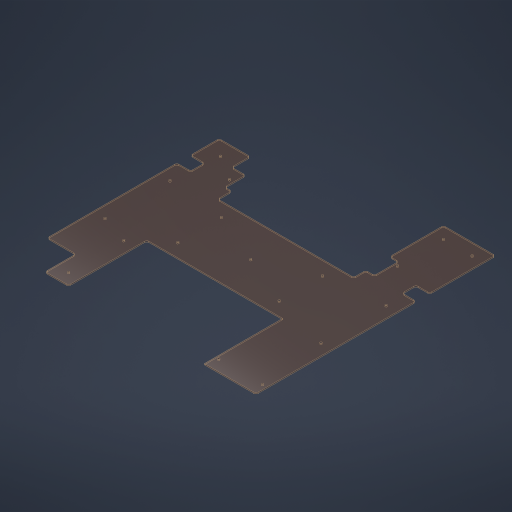
# Autodesk Inventor part: DB1-023
Saved by Autodesk Inventor 2023.4 (Build 274418000, 418)
## iProperties
Created: 2025-03-10
Part Number: DB1-023
Material: Polycarbonate, Smoke
Document SubType Name: Sheet Metal
Designer: brand
Density: 1.2 g/cm^3
Sheet Metal Rule: Default
Appearance: Polycarbonate - Smoked
Author: brand
Autodesk Inventor part; units mm, degrees
ref_plane "YZ Plane" through (0, 0, 0) normal (1, 0, 0) x (0, 1, 0)
ref_plane "XZ Plane" through (0, 0, 0) normal (0, 1, 0) x (-1, 0, 0)
ref_plane "XY Plane" through (0, 0, 0) normal (0, 0, 1) x (1, 0, 0)
sketch "Sketch1" plane through (0, 0, 0) normal (0, 1, 0) x (-1, 0, 0)
  line L0 (329.819, 329.819) -> (-329.819, 329.819)
  line L1 (-329.819, 329.819) -> (-329.819, -329.819)
  line L2 (-329.819, -329.819) -> (329.819, -329.819)
  line L3 (329.819, -329.819) -> (329.819, 329.819)
  line L4 (329.819, 329.819) -> (-329.819, -329.819) construction
  line L5 (-329.819, 329.819) -> (329.819, -329.819) construction
  line L6 (187.325, 329.819) -> (-187.325, 329.819) construction
  line L7 (-187.325, 329.819) -> (-187.325, 113.919)
  line L8 (-187.325, 113.919) -> (187.325, 113.919)
  line L9 (187.325, 113.919) -> (187.325, 329.819)
  line L10 (187.325, -329.819) -> (-187.325, -329.819) construction
  line L11 (-187.325, -329.819) -> (-187.325, -82.169)
  line L12 (-187.325, -82.169) -> (187.325, -82.169)
  line L13 (187.325, -82.169) -> (187.325, -329.819)
  point P0 (0, 0)
  point P1 (0, 329.819)
  point P2 (0, 329.819)
  point P3 (0, -329.819)
  point P4 (0, -329.819)
  point P5 (-187.325, 329.819)
  dimension "d0" = 659.638
  dimension "d1" = 659.638
  dimension "d3" = 215.9
  dimension "d4" = 247.65
  dimension "d5" = 374.65
  constraints: 28 end point, 6 midpoint, 6 parallel, 3 horizontal, 3 perpendicular, 2 coincident, 2 point on line, 1 collinear
  measures "d0" distance of L0.start L0.end
  measures "d1" distance of L2.end L0.start
  measures "d3" distance of L8.end L6.start
  measures "d4" distance of L12.end L10.start
  measures "d5" distance of L11.end L12.end
extrude "Extrusion1" add sketch "Sketch1" along normal mid plane 3.175 contours L3 L2 L13 L12 L11 L1 L0 L7 L8 L9
sketch "Sketch2" plane through (0, 1.5875, 0) normal (0, 1, 0) x (1, 0, 0)
  circle A0 centre (-283.3124, 275.8316) radius 34.925 construction
  line L0 (329.819, 329.819) -> (329.819, -329.819) construction
  line L1 (329.819, -329.819) -> (187.325, -329.819) construction
  line L2 (187.325, -329.819) -> (187.325, -113.919) construction
  line L3 (187.325, -113.919) -> (-187.325, -113.919) construction
  line L4 (-187.325, -113.919) -> (-187.325, -329.819) construction
  line L5 (-187.325, -329.819) -> (-329.819, -329.819) construction
  line L6 (-329.819, -329.819) -> (-329.819, 329.819) construction
  line L7 (-329.819, 329.819) -> (-187.325, 329.819) construction
  line L8 (-187.325, 329.819) -> (-187.325, 82.169) construction
  line L9 (-187.325, 82.169) -> (187.325, 82.169) construction
  line L10 (187.325, 82.169) -> (187.325, 329.819) construction
  line L11 (187.325, 329.819) -> (329.819, 329.819) construction
  line L12 (-187.325, 329.819) -> (-329.819, 329.819) construction
  line L13 (-329.819, 329.819) -> (-187.325, 329.819)
  line L14 (-187.325, 329.819) -> (-187.325, 228.219)
  line L15 (-187.325, 228.219) -> (-329.819, 228.219)
  line L16 (-329.819, 228.219) -> (-329.819, 329.819)
  line L17 (329.819, -329.819) -> (187.325, -329.819) construction
  line L18 (187.325, -113.919) -> (206.375, -113.919)
  line L19 (206.375, -113.919) -> (206.375, -329.819)
  line L20 (206.375, -329.819) -> (187.325, -329.819)
  line L21 (187.325, -329.819) -> (187.325, -113.919)
  line L22 (-329.819, 329.819) -> (-329.819, -329.819) construction
  line L23 (-329.819, 149.606) -> (-291.719, 149.606)
  line L24 (-291.719, 149.606) -> (-291.719, 111.506)
  line L25 (-291.719, 111.506) -> (-329.819, 111.506)
  line L26 (-329.819, 111.506) -> (-329.819, 149.606)
  line L27 (329.819, 149.606) -> (291.719, 149.606)
  line L28 (291.719, 149.606) -> (291.719, 111.506)
  line L29 (291.719, 111.506) -> (329.819, 111.506)
  line L30 (329.819, 111.506) -> (329.819, 149.606)
  line L31 (206.375, -113.919) -> (250.825, -113.919)
  line L32 (250.825, -113.919) -> (250.825, -266.319)
  line L33 (250.825, -266.319) -> (206.375, -266.319)
  line L34 (206.375, -266.319) -> (206.375, -113.919)
  line L35 (-187.325, 82.169) -> (-187.325, 329.819) construction
  line L36 (-187.325, 228.219) -> (-244.475, 228.219)
  line L37 (-244.475, 228.219) -> (-244.475, 177.419)
  line L38 (-244.475, 177.419) -> (-187.325, 177.419)
  line L39 (-187.325, 177.419) -> (-187.325, 228.219)
  circle A1 centre (-219.075, 209.169) radius 19.05 construction
  line L40 (-329.819, -329.819) -> (-187.325, -329.819) construction
  line L41 (-329.819, -329.819) -> (-187.325, -329.819)
  line L42 (-187.325, -329.819) -> (-187.325, -228.219)
  line L43 (-187.325, -228.219) -> (-329.819, -228.219)
  line L44 (-329.819, -228.219) -> (-329.819, -329.819)
  point P0 (0, 0)
  point P1 (-329.819, 130.556)
  dimension "d9" = 69.85
  dimension "d10" = 46.5066
  dimension "d11" = 53.9874
  dimension "d12" = 101.6
  dimension "d16" = 19.05
  dimension "d17" = 460.375
  dimension "d18" = 38.1
  dimension "d19" = 38.1
  dimension "d20" = 63.5
  dimension "d21" = 63.5
  dimension "d28" = 38.1
  dimension "d29" = 31.75
  dimension "d30" = 120.65
  dimension "d31" = 57.15
  dimension "d32" = 50.8
  dimension "d61" = 101.6
  constraints: 56 end point, 15 parallel, 7 horizontal, 7 perpendicular, 5 point on line, 2 centre point, 2 horizontal alignment, 1 midpoint
  measures "d9" diameter of A0
  measures "d10" distance from line of L16 A0.centre
  measures "d11" distance from line of L7 A0.centre
  measures "d12" distance of L13.end L14.end
  measures "d16" distance of L2.end L18.end
  measures "d17" distance from line of L5 point (-329.819, 130.556)
  measures "d18" distance of L23.end L24.end
  measures "d19" distance of L24.end L25.end
  measures "d20" distance between parallel lines of L2 L32
  measures "d21" distance between parallel lines of L1 L33
  measures "d28" diameter of A1
  measures "d29" distance from line of L35 A1.centre
  measures "d30" distance from line of L7 A1.centre
  measures "d31" distance of L37.end L38.end
  measures "d32" distance of L36.end L37.end
  measures "d61" distance of L43.end L5.end
extrude "Extrusion2" cut sketch "Sketch2" against normal through all contours L13 L14 L15 L16 | L39 L38 L37 L15 | L23 L24 L25 L26 | L30 L29 L28 L27
fillet "Fillet1" radius 5.715 20 edges at (-187.325, 0, 113.919) (329.819, 0, 329.819) (329.819, 0, -329.819) (187.325, 0, -329.819) (187.325, 0, -82.169) (-187.325, 0, -82.169) (-329.819, 0, 329.819) (-329.819, 0, -228.219) (-329.819, 0, -149.606) (-291.719, 0, -149.606) (-291.719, 0, -111.506) (-329.819, 0, -111.506) (291.719, 0, -149.606) (291.719, 0, -111.506) (329.819, 0, -111.506) (329.819, 0, -149.606) (-187.325, 0, -177.419) (-244.475, 0, -177.419) (-244.475, 0, -228.219) (-187.325, 0, 329.819)
sketch "Sketch4" plane through (0, 1.5875, 0) normal (0, 1, 0) x (1, 0, 0)
  arc A0 (324.104, -329.819) -> (329.819, -324.104) centre (324.104, -324.104) ccw construction
  line L0 (324.104, -329.819) -> (187.325, -329.819) construction
  line L1 (187.325, -113.919) -> (-181.61, -113.919) construction
  arc A1 (-181.61, -113.919) -> (-187.325, -119.634) centre (-181.61, -119.634) ccw construction
  line L2 (-187.325, -119.634) -> (-187.325, -324.104) construction
  arc A2 (-193.04, -329.819) -> (-187.325, -324.104) centre (-193.04, -324.104) ccw construction
  arc A3 (-329.819, -324.104) -> (-324.104, -329.819) centre (-324.104, -324.104) ccw construction
  line L3 (-329.819, -324.104) -> (-329.819, 105.791) construction
  arc A4 (-324.104, 111.506) -> (-329.819, 105.791) centre (-324.104, 105.791) ccw construction
  line L4 (-324.104, 111.506) -> (-297.434, 111.506) construction
  arc A5 (-297.434, 111.506) -> (-291.719, 117.221) centre (-297.434, 117.221) ccw construction
  line L5 (-291.719, 117.221) -> (-291.719, 143.891) construction
  arc A6 (-291.719, 143.891) -> (-297.434, 149.606) centre (-297.434, 143.891) ccw construction
  line L6 (-297.434, 149.606) -> (-324.104, 149.606) construction
  arc A7 (-329.819, 155.321) -> (-324.104, 149.606) centre (-324.104, 155.321) ccw construction
  line L7 (-329.819, 155.321) -> (-329.819, 222.504) construction
  arc A8 (-324.104, 228.219) -> (-329.819, 222.504) centre (-324.104, 222.504) ccw construction
  line L8 (-324.104, 228.219) -> (-250.19, 228.219) construction
  arc A9 (-244.475, 222.504) -> (-250.19, 228.219) centre (-250.19, 222.504) ccw construction
  line L9 (-244.475, 222.504) -> (-244.475, 183.134) construction
  arc A10 (-244.475, 183.134) -> (-238.76, 177.419) centre (-238.76, 183.134) ccw construction
  line L10 (-238.76, 177.419) -> (-193.04, 177.419) construction
  arc A11 (-187.325, 171.704) -> (-193.04, 177.419) centre (-193.04, 171.704) ccw construction
  line L11 (-187.325, 171.704) -> (-187.325, 87.884) construction
  arc A12 (-187.325, 87.884) -> (-181.61, 82.169) centre (-181.61, 87.884) ccw construction
  line L12 (-181.61, 82.169) -> (181.61, 82.169) construction
  arc A13 (181.61, 82.169) -> (187.325, 87.884) centre (181.61, 87.884) ccw construction
  line L13 (187.325, 87.884) -> (187.325, 324.104) construction
  arc A14 (193.04, 329.819) -> (187.325, 324.104) centre (193.04, 324.104) ccw construction
  line L14 (193.04, 329.819) -> (324.104, 329.819) construction
  arc A15 (329.819, 324.104) -> (324.104, 329.819) centre (324.104, 324.104) ccw construction
  line L15 (329.819, 324.104) -> (329.819, 155.321) construction
  arc A16 (324.104, 149.606) -> (329.819, 155.321) centre (324.104, 155.321) ccw construction
  line L16 (324.104, 149.606) -> (297.434, 149.606) construction
  arc A17 (297.434, 149.606) -> (291.719, 143.891) centre (297.434, 143.891) ccw construction
  line L17 (291.719, 143.891) -> (291.719, 117.221) construction
  arc A18 (291.719, 117.221) -> (297.434, 111.506) centre (297.434, 117.221) ccw construction
  line L18 (297.434, 111.506) -> (324.104, 111.506) construction
  arc A19 (329.819, 105.791) -> (324.104, 111.506) centre (324.104, 105.791) ccw construction
  line L19 (329.819, 105.791) -> (329.819, -324.104) construction
  line L20 (195.3895, -298.069) -> (316.0395, -298.069) construction
  line L21 (329.819, 105.791) -> (329.819, -324.104) construction
  line L22 (187.325, -113.919) -> (-181.61, -113.919) construction
  line L23 (2.8575, -113.919) -> (0, 82.169) construction
  line L24 (-324.104, 155.321) -> (-250.19, 222.504) construction
  line L25 (-298.069, 60.706) -> (-298.069, -298.069) construction
  line L26 (-193.04, -329.819) -> (-324.104, -329.819) projected
  line L27 (187.325, -329.819) -> (187.325, -113.919) projected
  point P0 (0, 0)
  point P1 (139.7, 44.069)
  point P2 (139.7, -75.819)
  point P3 (-139.7, 44.069)
  point P4 (-139.7, -75.819)
  point P5 (1.4288, -15.875)
  point P6 (298.069, 60.706)
  point P7 (298.069, 298.069)
  point P8 (219.075, 298.069)
  point P9 (-219.075, -145.669)
  point P10 (298.069, -118.6815)
  point P11 (-298.069, -118.6815)
  point P12 (-287.147, 188.9125)
  point P13 (193.9925, -298.069)
  point P14 (255.7145, -298.069)
  point P15 (255.7145, -329.819)
  point P16 (1.4288, -15.875)
  point P17 (-219.075, -298.069)
  point P18 (-287.147, 188.9125)
  point P19 (-219.075, 145.669)
  point P20 (-215.9, 177.419)
  point P21 (-298.069, -118.6815)
  point P22 (219.075, 171.069)
  dimension "d33" = 120.65
  dimension "d34" = 31.75
  dimension "d35" = 31.75
  dimension "d36" = 31.75
  dimension "d37" = 31.75
  dimension "d38" = 31.75
  dimension "d39" = 50.8
  dimension "d40" = 47.625
  dimension "d41" = 38.1
  dimension "d42" = 38.1
  dimension "d43" = 47.625
  dimension "d44" = 31.75
  dimension "d47" = 31.75
  dimension "d48" = 31.75
  dimension "d49" = 31.75
  dimension "d50" = 50.8
  dimension "d51" = 31.75
  dimension "d59" = 127
  dimension "d60" = 31.75
  constraints: 8 end point, 8 midpoint, 8 vertical alignment, 7 horizontal alignment, 3 coincident, 1 horizontal, 1 vertical
  measures "d33" distance of L20.end L20.start
  measures "d34" distance from line of L14 point (298.069, 298.069)
  measures "d35" distance from line of L15 point (298.069, 298.069)
  measures "d36" distance from line of L13 point (219.075, 298.069)
  measures "d37" distance from line of L14 point (219.075, 298.069)
  measures "d38" distance from line of L19 point (298.069, 60.706)
  measures "d39" distance from line of point (298.069, 60.706) L18
  measures "d40" distance from line of L13 point (139.7, 44.069)
  measures "d41" distance from line of L12 point (139.7, 44.069)
  measures "d42" distance from line of L1 point (139.7, -75.819)
  measures "d43" distance from line of L11 point (-139.7, 44.069)
  measures "d44" distance from line of L2 point (-219.075, -298.069)
  measures "d47" distance from line of L3 L25.end
  measures "d48" vertical distance of point (-219.075, 145.669) point (-215.9, 177.419)
  measures "d49" distance from line of L11 point (-219.075, 145.669)
  measures "d50" distance from line of L4 L25.start
  measures "d51" distance from line of L1 point (-219.075, -145.669)
  measures "d59" distance of point (219.075, 171.069) point (219.075, 298.069)
  measures "d60" distance from line of L26 point (-219.075, -298.069)
hole "Hole1" at (-298.069, 1.5875, 298.069) at (316.0395, 1.5875, 298.069) at (139.7, 1.5875, -44.069) at (139.7, 1.5875, 75.819) at (-139.7, 1.5875, -44.069) at (-139.7, 1.5875, 75.819) at (1.4288, 1.5875, 15.875) at (-298.069, 1.5875, -60.706) at (298.069, 1.5875, -60.706) at (298.069, 1.5875, -298.069) at (219.075, 1.5875, -298.069) at (-219.075, 1.5875, 145.669) at (195.3895, 1.5875, 298.069) at (298.069, 1.5875, 118.6815) at (-298.069, 1.5875, 118.6815) at (-287.147, 1.5875, -188.9125) at (-219.075, 1.5875, 298.069) at (-219.075, 1.5875, -145.669) at (219.075, 1.5875, -171.069) direction (0, -1, 0) diameter 5.1054 end through all clearance for "Flat Head Machine Screw (82)" size "#10" standard "Ansi Unified Screw Threads"
sketch "Sketch5" plane through (0, 1.5875, 0) normal (0, 1, 0) x (1, 0, 0)
  circle A0 centre (-219.075, 145.669) radius 2.5527 construction
  circle A1 centre (-287.147, 188.9125) radius 2.5527 construction
  circle A2 centre (298.069, -118.6815) radius 2.5527 construction
  circle A3 centre (-219.075, -145.669) radius 2.5527 construction
  circle A4 centre (298.069, 298.069) radius 2.5527 construction
  circle A5 centre (-298.069, 60.706) radius 2.5527 construction
  circle A6 centre (-139.7, -75.819) radius 2.5527 construction
  circle A7 centre (139.7, -75.819) radius 2.5527 construction
  circle A8 centre (316.0395, -298.069) radius 2.5527 construction
  circle A9 centre (-298.069, -298.069) radius 2.5527 construction
  circle A10 centre (139.7, 44.069) radius 2.5527 construction
  circle A11 centre (-139.7, 44.069) radius 2.5527 construction
  circle A12 centre (1.4288, -15.875) radius 2.5527 construction
  circle A13 centre (298.069, 60.706) radius 2.5527 construction
  circle A14 centre (219.075, 298.069) radius 2.5527 construction
  circle A15 centre (195.3895, -298.069) radius 2.5527 construction
  circle A16 centre (-298.069, -118.6815) radius 2.5527 construction
  circle A17 centre (-219.075, -298.069) radius 2.5527 construction
  circle A18 centre (219.075, 171.069) radius 2.5527 construction
  arc A19 (-181.61, -113.919) -> (-187.325, -119.634) centre (-181.61, -119.634) ccw construction
  line L0 (-187.325, -119.634) -> (-187.325, -324.104) construction
  arc A20 (-193.04, -329.819) -> (-187.325, -324.104) centre (-193.04, -324.104) ccw construction
  line L1 (-193.04, -329.819) -> (-324.104, -329.819) construction
  arc A21 (-329.819, -324.104) -> (-324.104, -329.819) centre (-324.104, -324.104) ccw construction
  line L2 (-329.819, -324.104) -> (-329.819, 105.791) construction
  arc A22 (-324.104, 111.506) -> (-329.819, 105.791) centre (-324.104, 105.791) ccw construction
  line L3 (-324.104, 111.506) -> (-297.434, 111.506) construction
  arc A23 (-297.434, 111.506) -> (-291.719, 117.221) centre (-297.434, 117.221) ccw construction
  line L4 (-291.719, 117.221) -> (-291.719, 143.891) construction
  arc A24 (-291.719, 143.891) -> (-297.434, 149.606) centre (-297.434, 143.891) ccw construction
  line L5 (-297.434, 149.606) -> (-324.104, 149.606) construction
  arc A25 (-329.819, 155.321) -> (-324.104, 149.606) centre (-324.104, 155.321) ccw construction
  line L6 (-329.819, 155.321) -> (-329.819, 222.504) construction
  arc A26 (-324.104, 228.219) -> (-329.819, 222.504) centre (-324.104, 222.504) ccw construction
  line L7 (-324.104, 228.219) -> (-250.19, 228.219) construction
  arc A27 (-244.475, 222.504) -> (-250.19, 228.219) centre (-250.19, 222.504) ccw construction
  line L8 (-244.475, 222.504) -> (-244.475, 183.134) construction
  arc A28 (-244.475, 183.134) -> (-238.76, 177.419) centre (-238.76, 183.134) ccw construction
  line L9 (-238.76, 177.419) -> (-193.04, 177.419) construction
  arc A29 (-187.325, 171.704) -> (-193.04, 177.419) centre (-193.04, 171.704) ccw construction
  line L10 (-187.325, 171.704) -> (-187.325, 87.884) construction
  arc A30 (-187.325, 87.884) -> (-181.61, 82.169) centre (-181.61, 87.884) ccw construction
  line L11 (-181.61, 82.169) -> (181.61, 82.169) construction
  arc A31 (181.61, 82.169) -> (187.325, 87.884) centre (181.61, 87.884) ccw construction
  line L12 (187.325, 87.884) -> (187.325, 324.104) construction
  arc A32 (193.04, 329.819) -> (187.325, 324.104) centre (193.04, 324.104) ccw construction
  line L13 (193.04, 329.819) -> (324.104, 329.819) construction
  arc A33 (329.819, 324.104) -> (324.104, 329.819) centre (324.104, 324.104) ccw construction
  line L14 (329.819, 324.104) -> (329.819, 155.321) construction
  arc A34 (324.104, 149.606) -> (329.819, 155.321) centre (324.104, 155.321) ccw construction
  line L15 (324.104, 149.606) -> (297.434, 149.606) construction
  arc A35 (297.434, 149.606) -> (291.719, 143.891) centre (297.434, 143.891) ccw construction
  line L16 (291.719, 143.891) -> (291.719, 117.221) construction
  arc A36 (291.719, 117.221) -> (297.434, 111.506) centre (297.434, 117.221) ccw construction
  line L17 (297.434, 111.506) -> (324.104, 111.506) construction
  arc A37 (329.819, 105.791) -> (324.104, 111.506) centre (324.104, 105.791) ccw construction
  line L18 (329.819, 105.791) -> (329.819, -324.104) construction
  arc A38 (324.104, -329.819) -> (329.819, -324.104) centre (324.104, -324.104) ccw construction
  line L19 (324.104, -329.819) -> (187.325, -329.819) construction
  line L20 (187.325, -329.819) -> (187.325, -113.919) construction
  line L21 (187.325, -113.919) -> (-181.61, -113.919) construction
  circle A39 centre (-296.2567, -289.5119) radius 34.925 construction
  line L22 (-251.8067, -245.0619) -> (-329.819, -245.0619)
  line L23 (-329.819, -245.0619) -> (-329.819, -329.819)
  line L24 (-329.819, -329.819) -> (-251.8067, -329.819)
  line L25 (-251.8067, -329.819) -> (-251.8067, -245.0619)
  line L26 (-324.104, -329.819) -> (-193.04, -329.819) construction
  line L27 (-187.325, 177.419) -> (-206.375, 177.419)
  line L28 (-206.375, 177.419) -> (-206.375, 120.269)
  line L29 (-206.375, 120.269) -> (-187.325, 120.269)
  line L30 (-187.325, 120.269) -> (-187.325, 177.419)
  line L31 (0, 82.169) -> (0, 0) construction
  line L32 (187.325, 171.704) -> (187.325, 87.884) construction
  line L33 (187.325, 177.419) -> (206.375, 177.419)
  line L34 (206.375, 177.419) -> (206.375, 120.269)
  line L35 (206.375, 120.269) -> (187.325, 120.269)
  line L36 (187.325, 120.269) -> (187.325, 177.419)
  line L37 (211.1375, 182.1815) -> (182.5625, 182.1815)
  line L38 (182.5625, 182.1815) -> (182.5625, 115.5065)
  line L39 (182.5625, 115.5065) -> (211.1375, 115.5065)
  line L40 (211.1375, 115.5065) -> (211.1375, 182.1815)
  point P0 (-296.2567, -254.5869)
  point P1 (-261.3317, -289.5119)
  dimension "d62" = 69.85
  dimension "d63" = 40.3071
  dimension "d64" = 33.5623
  dimension "d65" = 9.525
  dimension "d66" = 9.525
  dimension "d70" = 19.05
  dimension "d71" = 57.15
  dimension "d72" = 4.7625
  constraints: 36 end point, 5 point on line, 5 symmetric about line, 4 parallel, 2 horizontal, 2 perpendicular, 2 point on circle, 1 centre point, 1 horizontal alignment, 1 midpoint, 1 vertical, 1 vertical alignment, 3 other
  measures "d62" diameter of A39
  measures "d63" distance from line of L1 A39.centre
  measures "d64" distance from line of L2 A39.centre
  measures "d65" distance from line of L25 A39.end
  measures "d66" distance from line of L22 A39.start
  measures "d70" distance of L28.end L29.end
  measures "d71" distance of L27.end L28.end
  measures "d72" distance between parallel lines of L33 L37
extrude "Extrusion4" cut sketch "Sketch5" against normal through all contours L25 L24 L23 L22 | L30 L29 L28 L27 | L33 L34 L35 L36 | L40 L39 L38 L37
fillet "Fillet2" radius 5.715 10 edges at (-329.819, 0, 245.0619) (-251.8067, 0, 245.0619) (-251.8067, 0, 329.819) (-187.325, 0, -120.269) (-206.375, 0, -120.269) (-206.375, 0, -177.419) (187.325, 0, -115.5065) (211.1375, 0, -115.5065) (211.1375, 0, -182.1815) (187.325, 0, -182.1815)
equation "\"d19\" = d18"
equation "\"d35\" = d34"
equation "\"d36\" = d34"
equation "\"d37\" = d34"
equation "\"d38\" = d36"
equation "\"d42\" = d41"
equation "\"d44\" = d38"
equation "\"d47\" = d44"
equation "\"d49\" = d48"
equation "\"d57\" = Thickness"
equation "\"BendRadius\" = Thickness"
equation "\"BendReliefWidth\" = Thickness"
equation "\"BendReliefDepth\" = 0.5 * Thickness"
equation "\"CornerReliefSize\" = 4 * Thickness"
equation "\"MinimumRemnant\" = 2 * Thickness"
equation "\"TransitionRadius\" = BendRadius"
equation "\"JacobiRadiusSize\" = BendRadius"
equation "\"GapSize\" = Thickness"
equation "\"Thickness\" = 3.048"
body "Solid1"
